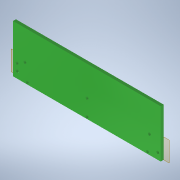
# Autodesk Inventor part: Poti_Sensor_PCB_
Saved by Autodesk Inventor 2022.2 (Build 262287010, 287A)
## iProperties
Created: 2024-07-23
Part Number: Poti_Sensor_PCB_
Material: Generisch
Document SubType Name: Modeling
Designer: ppovolni
Density: 1 g/cm^3
Appearance: Glatt - Waldgrün
Author: ppovolni
Autodesk Inventor part; units mm, degrees
ref_plane "YZ Plane" through (0, 0, 0) normal (1, 0, 0) x (0, 1, 0)
ref_plane "XZ Plane" through (0, 0, 0) normal (0, 1, 0) x (-1, 0, 0)
ref_plane "XY Plane" through (0, 0, 0) normal (0, 0, 1) x (1, 0, 0)
ref_plane "Arbeitsebene1" through (0, -3.9, 0.8) normal (0, -1, 0) x (-1, 0, 0)
ref_plane "Arbeitsebene2" through (0, 0, 0) normal (0, 0, 1) x (1, 0, 0)
sketch "Skizze2" plane through (0, 0, 0) normal (0, 0, 1) x (1, 0, 0)
  circle A0 centre (31.3386, -4.2236) radius 0.75
  circle A1 centre (-0.1614, -4.2236) radius 0.75
  circle A2 centre (-31.3614, -4.2236) radius 0.75
  circle A3 centre (-32.5696, 4.2222) radius 0.75
  circle A4 centre (-0.1614, 4.2222) radius 0.75
  circle A5 centre (32.3386, 4.2222) radius 0.75
  circle A6 centre (36.7419, -1.8509) radius 0.75
  circle A7 centre (-36.6614, -1.7266) radius 0.75
  circle A8 centre (-36.6614, 1.7763) radius 0.75
  line L0 (33.8386, 4.2222) -> (-46.1614, 4.2222) construction
  line L1 (-46.1614, 4.2222) -> (-46.1614, -4.2236) construction
  line L2 (-46.1614, -4.2236) -> (33.8386, -4.2236) construction
  line L3 (33.8386, -4.2236) -> (33.8386, 4.2222) construction
  line L4 (33.8386, -4.2236) -> (36.7419, -4.2236) construction
  line L5 (36.7419, -4.2236) -> (36.7419, 4.2222) construction
  line L6 (36.7419, 4.2222) -> (33.8386, 4.2222) construction
  line L7 (33.8386, 4.2222) -> (33.8386, -4.2236) construction
  line L8 (-46.1614, -4.2236) -> (-36.6614, -4.2236) construction
  line L9 (-36.6614, -4.2236) -> (-36.6614, 4.2222) construction
  line L10 (-36.6614, 4.2222) -> (-46.1614, 4.2222) construction
  line L11 (-46.1614, 4.2222) -> (-46.1614, -4.2236) construction
  line L12 (38.2419, -5.2236) -> (-38.7581, -5.2236)
  line L13 (-38.7581, -5.2236) -> (-38.7581, 19.7764)
  line L14 (-38.7581, 19.7764) -> (38.2419, 19.7764)
  line L15 (38.2419, 19.7764) -> (38.2419, -5.2236)
  point P0 (0, 0)
  dimension "d0" = 1.5
  dimension "d1" = 8.4458
  dimension "d2" = 80
  dimension "d3" = 33.8386
  dimension "d4" = 4.2222
  dimension "d5" = 2.5
  dimension "d6" = 1.5
  dimension "d7" = 13.5918
  dimension "d8" = 14.8
  dimension "d9" = 34
  dimension "d10" = 34
  dimension "d11" = 2.9033
  dimension "d12" = 2.3726
  dimension "d13" = 9.5
  dimension "d14" = 2.497
  dimension "d15" = 2.4459
  dimension "d16" = 25
  dimension "d17" = 77
  dimension "d18" = 1.5
  dimension "d19" = 1
  constraints: 32 end point, 10 point on line, 9 centre point, 8 equal radius, 8 parallel, 4 horizontal, 4 perpendicular
  measures "d0" diameter of A0
  measures "d1" distance of L2.end L0.start
  measures "d2" distance of L1.end L2.end
  measures "d3" distance from line of point (0, 0) L3
  measures "d4" distance from line of L0 point (0, 0)
  measures "d5" distance from line of L3 A0.centre
  measures "d6" distance from line of L3 A5.centre
  measures "d7" distance from line of L1 A3.centre
  measures "d8" distance from line of L1 A2.centre
  measures "d9" distance from line of L3 A4.centre
  measures "d10" distance from line of L3 A1.centre
  measures "d11" distance between parallel lines of L5 L3
  measures "d12" distance from line of L4 A6.centre
  measures "d13" distance between parallel lines of L1 L9
  measures "d14" distance from line of L2 A7.centre
  measures "d15" distance from line of L0 A8.centre
  measures "d16" distance of L14.end L12.start
  measures "d17" distance of L13.end L14.end
  measures "d18" distance from line of L15 A6.centre
  measures "d19" distance between parallel lines of L2 L12
extrude "Extrusion1" add sketch "Skizze2" along normal blind 1.5
